Autodesk Fusion 360 part; units mm, degrees
(part 2 of 2)
extrude "Extrude3" [suppressed]
ref_plane "WorkPlane3" through (170, 56, 6.5) normal (0, 0, 1) x (1, 0, 0)
extrude "Extrude4" [suppressed]
extrude "Extrude5" [suppressed]
named bodies: "PCB", "b 2.0", "m b", "m t", "2.0"
